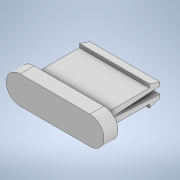
# Autodesk Inventor part: clip
Saved by Autodesk Inventor 2020.3 (Build 243373000, 373)
## iProperties
Created: 2020-08-14
Part Number: clip
Material: Generic
Document SubType Name: Modeling
Designer: aditk
Density: 1 g/cm^3
Appearance: Default
Author: aditk
Autodesk Inventor part; units mm, degrees
ref_plane "YZ Plane" through (0, 0, 0) normal (1, 0, 0) x (0, 1, 0)
ref_plane "XZ Plane" through (0, 0, 0) normal (0, 1, 0) x (-1, 0, 0)
ref_plane "XY Plane" through (0, 0, 0) normal (0, 0, 1) x (1, 0, 0)
sketch "Sketch1" plane through (0, 0, 0) normal (0, 0, 1) x (1, 0, 0)
  line L0 (-5, 0) -> (5, 0) construction
  line L1 (-5, -1) -> (5, -1)
  line L2 (5, 1) -> (-5, 1)
  arc A0 (-5, 1) -> (-5, -1) centre (-5, 0) ccw
  arc A1 (5, -1) -> (5, 1) centre (5, 0) ccw
  line L3 (-5, 0) -> (5, 0) construction
  line L4 (-5, -2) -> (5, -2)
  line L5 (5, 2) -> (-5, 2)
  arc A2 (-5, 2) -> (-5, -2) centre (-5, 0) ccw
  arc A3 (5, -2) -> (5, 2) centre (5, 0) ccw
  point P0 (0, 0)
  constraints: 16 end point, 8 point on circle, 8 tangent, 4 centre point, 3 equal length, 2 midpoint, 1 horizontal
extrude "Extrusion1" add sketch "Sketch1" along normal blind 2 contours A0 L2 A1 L1 | A2 L5 A3 L4
sketch "Sketch2" plane through (0, 0, 0) normal (0, 0, -1) x (-1, 0, 0)
  arc A0 (5, -2) -> (5, 2) centre (5, 0) ccw projected
  line L0 (-5, 0) -> (5, 0) construction
  line L1 (-5, -1) -> (5, -1)
  line L2 (5, 1) -> (-5, 1)
  arc A1 (-5, 1) -> (-5, -1) centre (-5, 0) ccw
  arc A2 (5, -1) -> (5, 1) centre (5, 0) ccw
  line L3 (5, 1) -> (5, -1)
  line L4 (-5, -1) -> (-5, 1)
  point P0 (0, 0)
  constraints: 12 end point, 4 point on circle, 4 tangent, 2 centre point, 2 parallel, 1 horizontal, 1 midpoint, 1 vertical
extrude "Extrusion2" add sketch "Sketch2" along normal blind 8 contours L4 L2 L3 L1
sketch "Sketch3" plane through (5, -1, 0) normal (1, 0, 0) x (0, 0, -1)
  line L0 (0, 2) -> (8, 2) projected
  line L1 (8, 2) -> (6.5, 2)
  line L2 (6.5, 2) -> (6.5, 2.5)
  line L3 (6.5, 2.5) -> (8, 2)
  line L4 (0, 0) -> (8, 0) projected
  line L5 (8, 0) -> (6.5, 0)
  line L6 (6.5, 0) -> (6.5, -0.5)
  line L7 (6.5, -0.5) -> (8, 0)
  point P0 (0, 1)
  dimension "d8" = 1.5
  dimension "d9" = 0.5
  dimension "d10" = 0.5
  constraints: 12 end point, 4 point on line, 1 perpendicular
  measures "d8" distance of L0.end L1.end
  measures "d9" distance of L1.end L2.end
  measures "d10" distance of L5.end L6.end
extrude "Extrusion3" add sketch "Sketch3" against normal up to surface (10 mm away)
sketch "Sketch4" plane through (5, -1, 0) normal (1, 0, 0) x (0, 0, -1)
  line L0 (8, 0) -> (8, 2) projected
  line L1 (8, 1) -> (8, 1.5)
  line L2 (8, 1.5) -> (0, 1)
  line L3 (8, 1) -> (8, 0.5)
  line L4 (8, 0.5) -> (0, 1)
  dimension "d13" = 0.5
  dimension "d14" = 0.5
  constraints: 8 end point, 2 point on line, 1 midpoint
  measures "d13" distance of L1.start L1.end
  measures "d14" distance of L1.start L3.end
extrude "Extrusion4" cut sketch "Sketch4" against normal through all
body "Solid1"
